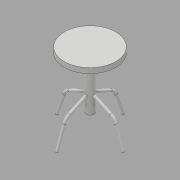
# Autodesk Inventor part: Chair_Orientation
Saved by Autodesk Inventor 2019.1 (Build 231200000, 200)
## iProperties
Created: 2018-10-29
Part Number: Chair_Orientation
Material: Generic
Document SubType Name: Modeling
Designer: t_gc
Density: 1 g/cm^3
Appearance: Default
Author: t_gc
Autodesk Inventor part; units mm, degrees
ref_plane "YZ Plane" through (0, 0, 0) normal (1, 0, 0) x (0, 1, 0)
ref_plane "XZ Plane" through (0, 0, 0) normal (0, 1, 0) x (-1, 0, 0)
sketch "Sketch1" plane through (0, 0, 0) normal (0, 0, 1) x (1, 0, 0)
  circle A0 centre (0, 0) radius 7.5
  dimension "d0" = 15
  constraints: 1 centre point, 1 coincident
  measures "d0" diameter of A0
extrude "Extrusion1" add sketch "Sketch1" along normal blind 100
sketch "Sketch2" plane through (0, 0, 100) normal (0, 0, 1) x (1, 0, 0)
  circle A0 centre (0, 0) radius 50
  dimension "d3" = 100
  constraints: 1 centre point, 1 coincident
  measures "d3" diameter of A0
extrude "Extrusion2" add sketch "Sketch2" along normal blind 10
sketch "Sketch3" plane through (0, 0, 0) normal (1, 0, 0) x (0, 1, 0)
  line L0 (-7.5, 0) -> (7.5, 0) projected
  line L1 (7.5, 0) -> (7.5, 100) projected
  arc A0 (50.3292, 5.6261) -> (40.3868, 16.5527) centre (32.5781, -0.5395) ccw
  line L2 (50.3292, 5.6261) -> (64.44, -35)
  line L3 (40.3868, 16.5527) -> (7.5, 31.5773)
  line L4 (7.5, 0) -> (7.5, 100) projected
  point P0 (0, 0)
  point P1 (0, 0)
  dimension "d14" = 64.44
  dimension "d15" = 35
  constraints: 4 end point, 2 point on circle, 2 tangent, 1 centre point, 1 coincident, 1 point on line
  measures "d14" horizontal distance of point (0, 0) L2.end
  measures "d15" vertical distance of point (0, 0) L2.end
ref_plane "Work Plane1" through (0, 64.44, -35) normal (0, 0.3281, -0.9446) x (-1, 0, 0)
sketch "Sketch4" plane through (0, 64.44, -35) normal (0, 0.3281, -0.9446) x (-1, 0, 0)
  circle A0 centre (0, 0) radius 2.5
  point P0 (0, -49.389)
  dimension "d7" = 5
  constraints: 1 centre point
  measures "d7" diameter of A0
sweep "Sweep1" add profiles "Sketch4" path "Sketch3" path curves L2 A0 L3
pattern_circular "Circular Pattern1" count 4 over 360 about axis through (0, 0, 0) along (0, 0, 1) of "Sweep1", "Extrusion1"
body "Solid1"
